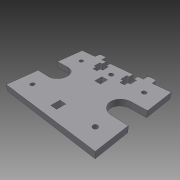
# Autodesk Inventor part: x_carryage_extruder_mount
Saved by Autodesk Inventor 2014 (Build 180170000, 170)
## iProperties
Created: 2014-02-23
Part Number: x_carryage_extruder_mount
Material: Generic
Document SubType Name: Modeling
Designer: buben
Density: 1 g/cm^3
Appearance: Default
Author: buben
Autodesk Inventor part; units mm, degrees
ref_plane "YZ Plane" through (0, 0, 0) normal (1, 0, 0) x (0, 1, 0)
ref_plane "XZ Plane" through (0, 0, 0) normal (0, 1, 0) x (-1, 0, 0)
ref_plane "XY Plane" through (0, 0, 0) normal (0, 0, 1) x (1, 0, 0)
sketch "Sketch1" plane through (0, 0, 0) normal (0, 0, 1) x (1, 0, 0)
  line L0 (0, 0) -> (92, 0)
  line L1 (92, 78) -> (0, 78)
  line L2 (0, 49) -> (13.5, 49)
  arc A0 (13.5, 29) -> (13.5, 49) centre (13.5, 39) ccw
  line L3 (13.5, 29) -> (0, 29)
  line L4 (92, 49) -> (78.5, 49)
  arc A1 (78.5, 49) -> (78.5, 29) centre (78.5, 39) ccw
  line L5 (78.5, 29) -> (92, 29)
  line L6 (0, 78) -> (0, 49)
  line L7 (0, 29) -> (0, 0)
  line L8 (92, 0) -> (92, 29)
  line L9 (92, 49) -> (92, 78)
  dimension "d0" = 92
  dimension "d1" = 20
  dimension "d2" = 78
  dimension "d3" = 39
  dimension "d11" = 65
  constraints: 20 end point, 8 perpendicular, 6 parallel, 5 collinear, 4 point on circle, 4 tangent, 2 centre point, 1 horizontal
  measures "d0" distance of L0.start L0.end
  measures "d1" distance between parallel lines of L3 L2
  measures "d2" distance of L0.start L1.end
  measures "d3" vertical distance of L0.start A0.centre
  measures "d11" distance of A1.centre A0.centre
extrude "Extrusion1" add sketch "Sketch1" along normal blind 6
sketch "Sketch2" plane through (0, 0, 6) normal (0, 0, 1) x (1, 0, 0)
  arc A0 (78.5, 49) -> (78.5, 29) centre (78.5, 39) ccw projected
  arc A1 (13.5, 29) -> (13.5, 49) centre (13.5, 39) ccw projected
  line L0 (13.5, 64) -> (78.5, 64) construction
  line L1 (78.5, 64) -> (78.5, 14) construction
  line L2 (78.5, 14) -> (13.5, 14) construction
  line L3 (13.5, 14) -> (13.5, 64) construction
  circle A2 centre (13.5, 64) radius 2.1
  circle A3 centre (13.5, 14) radius 2.1
  circle A4 centre (78.5, 14) radius 2.1
  circle A5 centre (78.5, 64) radius 2.1
  dimension "d7" = 4.2
  dimension "d8" = 50
  constraints: 8 end point, 4 centre point, 4 coincident, 3 equal radius, 3 midpoint, 2 parallel, 1 horizontal, 1 perpendicular
  measures "d7" diameter of A2
  measures "d8" distance of L2.end L0.start
extrude "Extrusion2" cut sketch "Sketch2" against normal blind 6
sketch "Sketch3" plane through (0, 0, 6) normal (0, 0, 1) x (1, 0, 0)
  line L0 (92, 78) -> (0, 78) projected
  line L1 (29.5, 78) -> (34, 78)
  line L2 (34, 61.7) -> (29.5, 61.7)
  line L3 (36.5, 73) -> (36.5, 65.7)
  line L4 (27, 65.7) -> (27, 73)
  line L5 (34, 78) -> (34, 73)
  line L6 (34, 65.7) -> (34, 61.7)
  line L7 (29.5, 61.7) -> (29.5, 65.7)
  line L8 (29.5, 73) -> (29.5, 78)
  line L9 (27, 73) -> (29.5, 73)
  line L10 (34, 73) -> (36.5, 73)
  line L11 (36.5, 65.7) -> (34, 65.7)
  line L12 (29.5, 65.7) -> (27, 65.7)
  line L13 (58, 78) -> (62.5, 78)
  line L14 (62.5, 61.7) -> (58, 61.7)
  line L15 (65, 73) -> (65, 65.7)
  line L16 (55.5, 65.7) -> (55.5, 73)
  line L17 (62.5, 78) -> (62.5, 73)
  line L18 (62.5, 65.7) -> (62.5, 61.7)
  line L19 (58, 61.7) -> (58, 65.7)
  line L20 (58, 73) -> (58, 78)
  line L21 (55.5, 73) -> (58, 73)
  line L22 (62.5, 73) -> (65, 73)
  line L23 (65, 65.7) -> (62.5, 65.7)
  line L24 (58, 65.7) -> (55.5, 65.7)
  line L25 (36.5, 69.35) -> (55.5, 69.35) construction
  point P0 (31.75, 61.7)
  point P1 (60.25, 61.7)
  point P2 (46, 69.35)
  point P3 (46, 78)
  dimension "d12" = 7.3
  dimension "d13" = 4
  dimension "d14" = 5
  dimension "d15" = 2.5
  dimension "d16" = 4.5
  dimension "d17" = 7.3
  dimension "d18" = 4
  dimension "d19" = 5
  dimension "d20" = 2.5
  dimension "d21" = 4.5
  dimension "d22" = 38
  constraints: 50 end point, 20 parallel, 12 collinear, 8 perpendicular, 6 horizontal, 6 midpoint, 1 vertical alignment
  measures "d12" distance of L4.start L4.end
  measures "d13" distance of L2.end L7.end
  measures "d14" distance of L8.start L1.start
  measures "d15" distance of L7.end L4.start
  measures "d16" distance of L2.start L2.end
  measures "d17" distance of L16.start L16.end
  measures "d18" distance of L14.end L24.start
  measures "d19" distance of L21.end L20.end
  measures "d20" distance of L24.start L16.start
  measures "d21" distance of L14.start L14.end
  measures "d22" distance between parallel lines of L15 L4
extrude "Extrusion3" cut sketch "Sketch3" against normal blind 6
sketch "Sketch4" plane through (0, 0, 6) normal (0, 0, 1) x (1, 0, 0)
  line L0 (29.5, 78) -> (0, 78) projected
  line L1 (92, 78) -> (62.5, 78) projected
  line L2 (62.5, 61.7) -> (58, 61.7) projected
  line L3 (34, 61.7) -> (29.5, 61.7) projected
  line L4 (16.25, 78) -> (24.25, 78)
  line L5 (24.25, 78) -> (24.25, 82)
  line L6 (22.25, 84) -> (18.25, 84)
  line L7 (16.25, 82) -> (16.25, 78)
  line L8 (67.75, 78) -> (75.75, 78)
  line L9 (75.75, 78) -> (75.75, 82)
  line L10 (73.75, 84) -> (69.75, 84)
  line L11 (67.75, 82) -> (67.75, 78)
  arc A0 (18.25, 84) -> (16.25, 82) centre (18.25, 82) ccw
  arc A1 (24.25, 82) -> (22.25, 84) centre (22.25, 82) ccw
  arc A2 (69.75, 84) -> (67.75, 82) centre (69.75, 82) ccw
  arc A3 (75.75, 82) -> (73.75, 84) centre (73.75, 82) ccw
  point P0 (31.75, 61.7)
  point P1 (60.25, 61.7)
  dimension "d25" = 2
  dimension "d26" = 8
  dimension "d27" = 8
  dimension "d28" = 7.5
  dimension "d29" = 7.5
  dimension "d30" = 6
  constraints: 16 end point, 8 point on circle, 8 tangent, 4 centre point, 4 parallel, 3 equal radius, 2 horizontal, 2 midpoint, 2 perpendicular, 2 point on line, 1 collinear
  measures "d25" radius of A0
  measures "d26" distance between parallel lines of L5 L7
  measures "d27" distance between parallel lines of L9 L11
  measures "d28" distance from line of point (60.25, 61.7) L11
  measures "d29" distance from line of point (31.75, 61.7) L5
  measures "d30" distance between parallel lines of L0 L6
extrude "Extrusion4" add sketch "Sketch4" against normal blind 6
sketch "Sketch5" plane through (0, 0, 6) normal (0, 0, 1) x (1, 0, 0)
  line L0 (0, 0) -> (92, 0) projected
  line L1 (58, 78) -> (34, 78) projected
  line L2 (43, 58) -> (49, 58)
  line L3 (49, 58) -> (49, 50)
  line L4 (49, 50) -> (43, 50)
  line L5 (43, 50) -> (43, 58)
  line L6 (43, 16) -> (49, 16)
  line L7 (49, 16) -> (49, 8)
  line L8 (49, 8) -> (43, 8)
  line L9 (43, 8) -> (43, 16)
  point P0 (46, 0)
  point P1 (46, 8)
  dimension "d33" = 6
  dimension "d34" = 8
  dimension "d35" = 20
  dimension "d36" = 8
  constraints: 16 end point, 4 parallel, 3 collinear, 2 horizontal, 2 midpoint, 2 perpendicular, 1 vertical alignment
  measures "d33" distance of L2.start L2.end
  measures "d34" distance of L4.end L2.start
  measures "d35" distance between parallel lines of L1 L2
  measures "d36" distance between parallel lines of L0 L8
extrude "Extrusion5" cut sketch "Sketch5" against normal blind 6
sketch "Sketch6" plane through (0, 0, 6) normal (0, 0, 1) x (1, 0, 0)
  line L0 (43, 58) -> (49, 58) projected
  line L1 (58, 78) -> (34, 78) projected
  circle A0 centre (46, 65.5) radius 2.25
  point P0 (46, 58)
  dimension "d39" = 4.5
  dimension "d40" = 12.5
  constraints: 1 centre point, 1 midpoint, 1 vertical alignment
  measures "d39" diameter of A0
  measures "d40" distance from line of L1 A0.centre
extrude "Extrusion6" cut sketch "Sketch6" against normal through all
equation "\"d3\" = 0.5 * d2"
body "Solid1"
